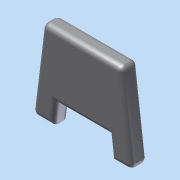
# Autodesk Inventor part: RUCBase
Saved by Autodesk Inventor 2011 SP1 (Build 150282100, 282)
## iProperties
Created: 2011-08-15
Part Number: RUCBase
Document SubType Name: Modeling
Designer: dgitz
Density: 1 g/cm^3
Author: dgitz
Autodesk Inventor part; units mm, degrees
ref_plane "YZ Plane" through (0, 0, 0) normal (1, 0, 0) x (0, 1, 0)
ref_plane "XZ Plane" through (0, 0, 0) normal (0, 1, 0) x (-1, 0, 0)
ref_plane "XY Plane" through (0, 0, 0) normal (0, 0, 1) x (1, 0, 0)
sketch "Sketch1" plane through (0, 0, 0) normal (0, 0, 1) x (1, 0, 0)
  line L0 (-34.134, 108.6265) -> (-59.534, -94.5735)
  line L1 (-59.534, -94.5735) -> (-8.734, -94.5735)
  line L2 (-8.734, -94.5735) -> (-2.384, -43.7735)
  line L3 (-2.384, -43.7735) -> (124.616, -43.7735)
  line L4 (124.616, -43.7735) -> (130.966, -94.5735)
  line L5 (130.966, -94.5735) -> (181.766, -94.5735)
  line L6 (181.766, -94.5735) -> (156.366, 108.6265)
  line L7 (156.366, 108.6265) -> (-34.134, 108.6265)
  point P0 (0, 0)
  dimension "d0" = 50.8
  dimension "d5" = 241.3
  dimension "d6" = 50.8
  dimension "d7" = 203.2
  dimension "d8" = 190.5
  dimension "d12" = 97.125
  dimension "d13" = 97.125
  constraints: 16 end point, 3 equal length, 3 horizontal, 3 parallel
  measures "d0" distance of L1.end L0.end
  measures "d5" distance of L5.end L0.end
  measures "d6" distance between parallel lines of L3 L1
  measures "d7" distance between parallel lines of L7 L1
  measures "d8" distance of L6.end L0.start
  measures "d12" angle of L0 L7
  measures "d13" angle of L6 L7
extrude "Extrusion1" add sketch "Sketch1" along normal blind 38.1
fillet "Fillet1" radius 12.7 20 edges at (61.116, 108.6265, 38.1) (-46.834, 7.0265, 38.1) (-34.134, -94.5735, 38.1) (-5.559, -69.1735, 38.1) (61.116, -43.7735, 38.1) (127.791, -69.1735, 38.1) (156.366, -94.5735, 38.1) (169.066, 7.0265, 38.1) (61.116, 108.6265, 0) (-46.834, 7.0265, 0) (-34.134, -94.5735, 0) (-5.559, -69.1735, 0) (61.116, -43.7735, 0) (127.791, -69.1735, 0) (156.366, -94.5735, 0) (169.066, 7.0265, 0) (156.366, 108.6265, 19.05) (181.766, -94.5735, 19.05) (-34.134, 108.6265, 19.05) (-59.534, -94.5735, 19.05)
body "Solid1"
